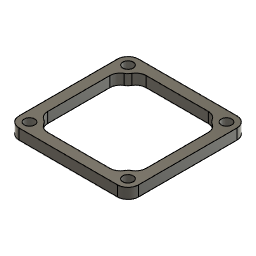
Spacer v1 (Autodesk Fusion 360 design; units mm, degrees)
Autodesk Fusion 360 part; units mm, degrees
sketch "Sketch1" plane through (0, 0, 0) normal (0, 1, 0) x (1, 0, 0)
  circle A0 centre (0, 0) radius 1.5
  circle A1 centre (-28.2, 0) radius 1.5
  circle A2 centre (-28.2, 28.2) radius 1.5
  circle A3 centre (0, 28.2) radius 1.5
  line L0 (-28.2, 31.2) -> (0, 31.2)
  line L1 (3, 28.2) -> (3, 0)
  line L2 (0, -3) -> (-28.2, -3)
  line L3 (-31.2, 0) -> (-31.2, 28.2)
  line L4 (-28.2, 23.0038) -> (-28.2, 5.1962)
  line L5 (-23.0038, 0) -> (-5.1962, 0)
  line L6 (0, 23.0038) -> (0, 5.1962)
  line L7 (-5.1962, 28.2) -> (-23.0038, 28.2)
  arc A4 (-28.2, 31.2) -> (-31.2, 28.2) centre (-28.2, 28.2) ccw
  arc A5 (-26.7, 25.6019) -> (-25.6019, 26.7) centre (-28.2, 28.2) ccw
  arc A6 (-31.2, 0) -> (-28.2, -3) centre (-28.2, 0) ccw
  arc A7 (-25.6019, 1.5) -> (-26.7, 2.5981) centre (-28.2, 0) ccw
  arc A8 (0, -3) -> (3, 0) centre (0, 0) ccw
  arc A9 (-1.5, 2.5981) -> (-2.5981, 1.5) centre (0, 0) ccw
  arc A10 (3, 28.2) -> (0, 31.2) centre (0, 28.2) ccw
  arc A11 (-2.5981, 26.7) -> (-1.5, 25.6019) centre (0, 28.2) ccw
  arc A12 (-26.7, 25.6019) -> (-28.2, 23.0038) centre (-25.2, 23.0038) ccw
  arc A13 (-23.0038, 28.2) -> (-25.6019, 26.7) centre (-23.0038, 25.2) ccw
  arc A14 (-28.2, 5.1962) -> (-26.7, 2.5981) centre (-25.2, 5.1962) ccw
  arc A15 (-25.6019, 1.5) -> (-23.0038, 0) centre (-23.0038, 3) ccw
  arc A16 (-5.1962, 0) -> (-2.5981, 1.5) centre (-5.1962, 3) ccw
  arc A17 (-1.5, 2.5981) -> (0, 5.1962) centre (-3, 5.1962) ccw
  arc A18 (0, 23.0038) -> (-1.5, 25.6019) centre (-3, 23.0038) ccw
  arc A19 (-2.5981, 26.7) -> (-5.1962, 28.2) centre (-5.1962, 25.2) ccw
  dimension "d1" = 28.2
  dimension "d2" = 28.2
  dimension "d3" = 3
  dimension "d4" = 3
  dimension "d5" = 3
  dimension "d6" = 3
  dimension "d7" = 6
  dimension "d8" = 6
  dimension "d9" = 6
  dimension "d10" = 6
  dimension "d11" = 3
  constraint coincident A0.centre A8.centre
  constraint concentric A2 A4
  constraint concentric A1 A6
  constraint concentric A0 A8
  constraint concentric A3 A10
  constraint tangent L0 A10
  constraint horizontal L0
  constraint tangent L1 A8
  constraint perpendicular L0 L1
  constraint tangent L2 A6
  constraint perpendicular L1 L2
  constraint tangent L3 A4
  constraint perpendicular L2 L3
  constraint vertical L4
  constraint perpendicular L4 L5
  constraint perpendicular L5 L6
  constraint perpendicular L6 L7
  constraint concentric A4 A5
  constraint concentric A6 A7
  constraint concentric A8 A9
  constraint concentric A10 A11
  constraint tangent L4 A12
  constraint tangent A5 A12
  constraint tangent L7 A13
  constraint tangent A5 A13
  constraint equal A12 A13
  constraint tangent L4 A14
  constraint tangent A7 A14
  constraint equal A12 A14
  constraint tangent L5 A15
  constraint tangent A7 A15
  constraint equal A12 A15
  constraint tangent L5 A16
  constraint tangent A9 A16
  constraint equal A12 A16
  constraint tangent L6 A17
  constraint tangent A9 A17
  constraint equal A12 A17
  constraint tangent L6 A18
  constraint tangent A11 A18
  constraint equal A12 A18
  constraint tangent L7 A19
  constraint tangent A11 A19
  constraint equal A12 A19
  measures "d1" distance of A0.centre A1.centre
  measures "d2" distance of A0.centre A3.centre
  measures "d3" diameter of A0
  measures "d4" diameter of A1
  measures "d5" diameter of A2
  measures "d6" diameter of A3
  measures "d7" diameter of A4
  measures "d8" diameter of A6
  measures "d9" diameter of A8
  measures "d10" diameter of A10
  measures "d11" radius of A12
extrude "Extrude1" add sketch "Sketch1" along normal blind 3
